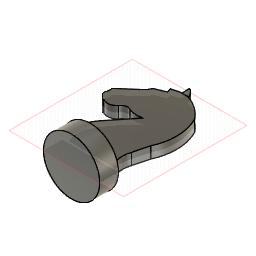
Knight2 (Autodesk Fusion 360 design; units mm, degrees)
Autodesk Fusion 360 part; units mm, degrees
sketch "Base" plane through (0, 0, 0) normal (0, 0, 1) x (1, 0, 0)
  line L0 (1.35, -11.2) -> (8.7, -11.2)
  line L1 (8.7, -11.2) -> (8.7, -16.1)
  line L2 (8.7, -16.1) -> (1.35, -16.1)
  line L3 (1.35, -16.1) -> (1.35, -11.2)
  line L4 (1.35, -11.2) -> (1.35, -16.5) construction
  constraint horizontal L0
  constraint vertical L1
  constraint horizontal L2
  constraint vertical L3
  constraint perpendicular L2 L4
revolve "Revolve1" add sketch "Base" angle 360 about axis through (1.35, -11.2, 0) along (0, -1, 0)
sketch "Sketch5" plane through (0, 0, 0) normal (0, 0, 1) x (1, 0, 0)
  line L0 (-3.8612, -3.6216) -> (1.2602, 2.7884)
  arc A0 (-2.4491, 2.9542) -> (-4.7968, 2.2709) centre (-3.3362, 1.6273) ccw
  arc A1 (-8.56, 1.8217) -> (-8.1023, 1.7795) centre (-8.3154, 1.9715) ccw
  arc A2 (-8.1023, 1.7795) -> (-4.7968, 2.2709) centre (-6.7484, 4.0355) ccw
  line L1 (-8.4888, 1.7431) -> (-9.6537, 3.0304)
  arc A3 (-9.5649, 4.0683) -> (-9.6537, 3.0304) centre (-8.6269, 3.4652) ccw
  line L2 (-9.5649, 4.0683) -> (-9.5, 4.9)
  arc A4 (-8.7221, 5.7752) -> (-9.5, 4.9) centre (-8.9, 5.15) ccw
  line L3 (-9.1971, 5.7281) -> (-5.657, 8.7735)
  arc A5 (-2.8723, 3.1545) -> (1.2602, 2.7884) centre (-0.3699, 7.8942) ccw
  line L4 (-3.8561, -11.9399) -> (7.9881, -11.9399)
  arc A6 (-3.8612, -3.6216) -> (-3.8561, -11.9399) centre (1.0426, -7.7778) ccw
  line L5 (-5.657, 8.7735) -> (-4.7, 9.7)
  line L6 (-4.7, 9.7) -> (-4.2, 10.7)
  line L7 (-4.2, 10.7) -> (-1.5, 11.8)
  line L8 (-1.5, 11.8) -> (-1.8, 12.9)
  line L9 (-1.8, 12.9) -> (0.0589, 13.407)
  line L10 (0.1583, 14.0219) -> (0.05, 16.1)
  arc A7 (0.0589, 13.407) -> (0.1571, 14.0443) centre (-1.3706, 13.9535) ccw
  arc A8 (2.2064, 13.4396) -> (0.05, 16.1) centre (-2.8988, 11.5057) ccw
  arc A9 (8.1474, 9.2996) -> (2.2064, 13.4396) centre (-1.7746, 1.394) ccw
  line L11 (8.5157, -2.5354) -> (7.2902, -7.2588)
  arc A10 (0.4921, 15.7841) -> (0.0594, 15.92) centre (-3.7578, 3.0059) ccw
  arc A11 (8.5157, -2.5354) -> (8.1474, 9.2996) centre (-3.7578, 3.0059) ccw
  arc A12 (7.4885, -6.4944) -> (7.9881, -11.9399) centre (14.1451, -8.6294) ccw
  line L12 (2.2064, 13.4396) -> (0.0589, 13.407)
  constraint coincident A0.start A5
  constraint coincident L1 A1.start
  constraint coincident A1 L1.start
  constraint coincident A4 L3.start
  constraint coincident A0 A5.start
  constraint horizontal L4
  constraint perpendicular L8 L9
  constraint coincident L10.start A7
  constraint coincident L10 A7.end
  constraint coincident A8 A10.start
  constraint coincident L11.start A10
  constraint coincident L10 A10.end
  constraint concentric A10 A11
  constraint coincident L11.end A12
  constraint coincident L11 A12.start
extrude "Extrude1" add sketch "Sketch5" along normal mid plane 3 contours L0 A0 A1 A2 L1 A3 L2 A4 L3 A5 L4 A6 L5 L6 L7 L8 L9 A9 L11 A11 A12 L12
extrude "Extrude2" add sketch "Sketch5" along normal mid plane 2 contours L10 A7 A8 A10 L12
